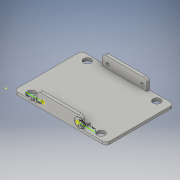
# Autodesk Inventor part: track guide u channel
Saved by Autodesk Inventor 2016 (Build 200138000, 138)
## iProperties
Created: 2015-10-31
Part Number: track guide u channel
Material: Generic
Document SubType Name: Modeling
Designer: Delta
Density: 1 g/cm^3
Appearance: Default
Author: Delta
Autodesk Inventor part; units mm, degrees
ref_plane "YZ Plane" through (0, 0, 0) normal (1, 0, 0) x (0, 1, 0)
ref_plane "XZ Plane" through (0, 0, 0) normal (0, 1, 0) x (-1, 0, 0)
ref_plane "XY Plane" through (0, 0, 0) normal (0, 0, 1) x (1, 0, 0)
sketch "Sketch1" plane through (0, 0, 0) normal (0, 0, 1) x (1, 0, 0)
  line L0 (0, 0) -> (101.6, 0)
  line L1 (101.6, 0) -> (101.6, 12.7)
  line L2 (101.6, 12.7) -> (0, 12.7)
  line L3 (0, 12.7) -> (0, 0)
  dimension "d0" = 101.6
  dimension "d1" = 12.7
  constraints: 8 end point, 2 parallel, 1 horizontal, 1 perpendicular
  measures "d0" distance of L2.end L1.end
  measures "d1" distance of L1.end L0.end
extrude "Extrusion1" add sketch "Sketch1" along normal blind 2.54
sketch "Sketch2" plane through (0, 0, 0) normal (0, 0, -1) x (-1, 0, 0)
  line L0 (-101.6, 0) -> (-101.6, 12.7) projected
  line L1 (0, 0) -> (-101.6, 0)
  line L2 (-101.6, 0) -> (-101.6, 2.54)
  line L3 (-101.6, 2.54) -> (0, 2.54)
  line L4 (0, 2.54) -> (0, 0)
  dimension "d4" = 2.54
  constraints: 8 end point, 2 parallel, 1 horizontal, 1 perpendicular, 1 point on line
  measures "d4" distance of L1.end L2.end
extrude "Extrusion2" add sketch "Sketch2" along normal blind 58.42
sketch "Sketch3" plane through (0, 0, -58.42) normal (0, 0, -1) x (-1, 0, 0)
  line L0 (-101.6, 12.7) -> (0, 12.7) projected
  line L1 (0, 0) -> (-101.6, 0)
  line L2 (-101.6, 0) -> (-101.6, 12.7)
  line L3 (-101.6, 12.7) -> (0, 12.7)
  line L4 (0, 12.7) -> (0, 0)
  dimension "d19" = 101.6
  constraints: 8 end point, 2 parallel, 1 horizontal, 1 perpendicular
  measures "d19" distance of L0.start L0.end
extrude "Extrusion3" add sketch "Sketch3" along normal blind 2.54
sketch "Sketch4" plane through (0, 0, 2.54) normal (0, 0, 1) x (1, 0, 0)
  line L0 (101.6, 12.7) -> (0, 12.7) projected
  line L1 (101.6, 0) -> (101.6, 12.7) projected
  point P0 (0, 0)
  point P1 (67.056, 6.35)
  point P2 (34.544, 6.35)
  dimension "d9" = 32.512
  dimension "d10" = 6.35
  dimension "d11" = 6.35
  dimension "d20" = 34.544
  measures "d9" distance of point (34.544, 6.35) point (67.056, 6.35)
  measures "d10" distance from line of L0 point (67.056, 6.35)
  measures "d11" distance from line of L0 point (34.544, 6.35)
  measures "d20" distance from line of point (67.056, 6.35) L1
hole "Hole1" at (67.056, 6.35, 2.54) at (34.544, 6.35, 2.54) direction (0, 0, -1) diameter 2.9972 end through all
sketch "Sketch5" plane through (0, 0, 2.54) normal (0, -1, 0) x (1, 0, 0)
  line L0 (101.6, -63.5) -> (101.6, 0) projected
  line L1 (0, 0) -> (101.6, 0) projected
  line L2 (0, 0) -> (0, -63.5) projected
  line L3 (101.6, -63.5) -> (0, -63.5) projected
  point P0 (0, -2.54)
  point P1 (83.4898, -5.5372)
  point P2 (18.288, -5.5372)
  point P3 (18.288, -57.9628)
  point P4 (83.4898, -57.9628)
  dimension "d21" = 18.1102
  dimension "d22" = 5.5372
  dimension "d23" = 5.5372
  dimension "d24" = 18.288
  dimension "d25" = 18.1102
  dimension "d26" = 5.5372
  dimension "d27" = 5.5372
  dimension "d28" = 18.288
  measures "d21" distance from line of L0 point (83.49, -5.537)
  measures "d22" distance from line of L1 point (83.49, -5.537)
  measures "d23" distance from line of L1 point (18.288, -5.537)
  measures "d24" distance from line of L2 point (18.288, -5.537)
  measures "d25" distance from line of L0 point (83.49, -57.963)
  measures "d26" distance from line of L3 point (83.49, -57.963)
  measures "d27" distance from line of L3 point (18.288, -57.963)
  measures "d28" distance from line of L2 point (18.288, -57.963)
hole "Hole2" at (83.4898, 0, -2.9972) at (18.288, 0, -2.9972) at (18.288, 0, -55.4228) at (83.4898, 0, -55.4228) direction (0, 1, 0) diameter 7.112 end through all
sketch "Sketch6" plane through (0, 0, 2.54) normal (0, 0, 1) x (1, 0, 0)
  circle A0 centre (34.544, 6.35) radius 1.4986 projected
  line L0 (33.0454, 6.35) -> (18.288, 6.35)
  circle A1 centre (67.056, 6.35) radius 1.4986 projected
  line L1 (68.5546, 6.35) -> (83.4898, 6.35)
  line L2 (68.5546, 6.35) -> (83.4898, 6.35) construction
  point P0 (0, 0)
  dimension "d36" = 14.7574
  dimension "d37" = 14.9352
  dimension "d38" = 0
  constraints: 6 end point, 3 horizontal, 2 horizontal alignment, 1 collinear, 2 other
  measures "d36" distance of L0.start L0.end
  measures "d37" distance of L1.start L1.end
  measures "d38" distance between parallel lines of L1 L2
sketch "Sketch8" plane through (0, 0, -60.96) normal (0, 0, -1) x (-1, 0, 0)
  line L0 (0, 0) -> (0, 2.54)
  line L1 (0, 0) -> (0, 12.7) projected
  line L2 (0, 12.7) -> (-29.211, 12.7)
  line L3 (-29.211, 12.7) -> (-29.211, 2.54)
  line L4 (-29.211, 2.54) -> (0, 2.54)
  line L5 (0, 2.54) -> (0, 12.7)
  dimension "d39" = 2.54
  constraints: 10 end point, 2 parallel, 1 horizontal, 1 perpendicular, 1 point on line
  measures "d39" distance of L0.start L0.end
extrude "Extrusion4" cut sketch "Sketch8" against normal through all
sketch "Sketch9" plane through (0, 0, 2.54) normal (0, -1, 0) x (1, 0, 0)
  line L0 (0, -63.5) -> (29.211, -63.5) projected
  line L1 (0, 0) -> (7.62, 0)
  line L2 (7.62, 0) -> (7.62, -63.5)
  line L3 (7.62, -63.5) -> (0, -63.5)
  line L4 (0, -63.5) -> (0, 0)
  line L5 (101.6, -2.54) -> (101.6, 0) projected
  line L6 (29.211, -63.5) -> (101.6, -63.5) projected
  line L7 (101.6, 0) -> (93.98, 0)
  line L8 (93.98, 0) -> (93.98, -63.5)
  line L9 (93.98, -63.5) -> (101.6, -63.5)
  line L10 (101.6, -63.5) -> (101.6, 0)
  point P0 (0, -2.54)
  dimension "d42" = 7.62
  dimension "d43" = 7.62
  constraints: 16 end point, 4 parallel, 2 horizontal, 2 perpendicular, 2 point on line
  measures "d42" distance of L2.end L3.end
  measures "d43" distance of L9.end L8.end
extrude "Extrusion5" cut sketch "Sketch9" against normal blind 25.4
sketch "Sketch10" plane through (0, 0, 2.54) normal (0, 0, 1) x (1, 0, 0)
  line L0 (7.62, 0) -> (93.98, 0) projected
  line L1 (93.98, 0) -> (93.98, 2.54)
  line L2 (93.98, 12.7) -> (29.211, 12.7) projected
  line L3 (93.98, 2.54) -> (71.12, 2.54)
  line L4 (71.12, 2.54) -> (71.12, 12.7)
  line L5 (71.12, 12.7) -> (93.98, 12.7)
  line L6 (93.98, 12.7) -> (93.98, 2.54)
  point P0 (0, 0)
  dimension "d46" = 2.54
  dimension "d47" = 22.86
  constraints: 10 end point, 2 parallel, 1 horizontal, 1 perpendicular, 1 point on line, 1 vertical
  measures "d46" distance of L0.end L1.end
  measures "d47" distance of L4.end L5.end
extrude "Extrusion6" cut sketch "Sketch10" against normal through all
fillet "Fillet1" radius 3.175 8 edges at (71.12, 12.7, 1.27) (29.211, 12.7, 1.27) (7.62, 1.27, -60.96) (7.62, 1.27, 2.54) (29.211, 12.7, -59.69) (71.12, 12.7, -59.69) (93.98, 1.27, -60.96) (93.98, 1.27, 2.54)
equation "\"d11\" = d10"
equation "\"d23\" = d22"
equation "\"d25\" = d21"
equation "\"d26\" = d22"
equation "\"d27\" = d22"
equation "\"d28\" = d24"
body "Solid1"
